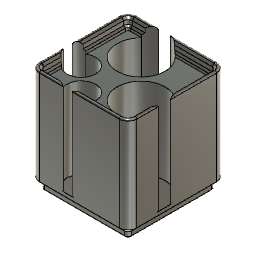
Gridfinity CR2032 + LR44 Holder (Autodesk Fusion 360 design; units mm, degrees)
Autodesk Fusion 360 part; units mm, degrees
sketch "Sketch1" plane through (0, 0, 0) normal (0, 0, 1) x (1, 0, 0) in component "Blank Storage"
  line L0 (0, 42) -> (42, 42)
  line L1 (42, 42) -> (42, 0)
  line L2 (42, 0) -> (0, 0)
  line L3 (0, 0) -> (0, 42)
  line L4 (0, 42) -> (42, 0) construction
  line L5 (42, 21) -> (0, 21) construction
  line L6 (42, 14.5) -> (0, 14.5)
  line L7 (42, 27.5) -> (0, 27.5)
  line L8 (27.5, 42) -> (27.5, 0)
  line L9 (14.5, 42) -> (14.5, 0)
  line L10 (14.5, 14.5) -> (0, 0) construction
  circle A0 centre (8, 8) radius 1.5
  circle A1 centre (34, 8) radius 1.5
  circle A2 centre (34, 34) radius 1.5
  circle A3 centre (8, 34) radius 1.5
  circle A4 centre (8, 8) radius 3.25
  circle A5 centre (34, 8) radius 3.25
  circle A6 centre (34, 34) radius 3.25
  circle A7 centre (8, 34) radius 3.25
  point P0 (21, 21)
  dimension "d1" = 42
  dimension "d2" = 42
  dimension "d65" = 13
  dimension "d67" = 90
  dimension "d69" = 3
  dimension "d71" = 360
  dimension "d80" = 6.5
  dimension "d85" = 8
  constraint horizontal L0
  constraint perpendicular L0 L1
  constraint parallel L0 L2
  constraint parallel L1 L3
  constraint coincident L2.end L3.start
  constraint midpoint L1 L5.start
  constraint midpoint L3 L5.end
  constraint coincident L1 L6.start
  constraint coincident L3 L6.end
  constraint perpendicular L3 L6
  constraint symmetric L5 L6.start L7.start
  constraint symmetric L5 L6.end L7.end
  constraint midpoint L4 P0
  constraint coincident L9 L10.start
  constraint coincident L6 L10.start
  constraint concentric A0 A4
  constraint coincident L10 A0.centre
  measures "d1" distance of L1.end L2.end
  measures "d2" distance of L0.end L1.end
  measures "d65" distance of L6 L7
  measures "d69" diameter of A0
  measures "d80" diameter of A4
  measures "d85" distance of L2 A0.centre
extrude "Extrude1" add sketch "Sketch1" along normal blind 5 contours L0 L3 L7 L9 | L0 L7 L8 L9 | L3 L6 L7 L9 | L0 L1 L7 L8 | L6 L7 L8 L9 | L2 L3 L6 L9 | L1 L6 L7 L8 | L2 L6 L8 L9 | L1 L2 L6 L8 | A0 | A1 | A2 | A3 | A4 | A5 | A6 | A7 makes body 1 in component "Blank Storage"
ref_plane "WorkPlane1" through (21, 21, 2.5) normal (0, -1, 0) x (1, 0, 0) in component "Blank Storage"
sketch "Sketch2" plane through (0, 21, 0) normal (0, -1, 0) x (1, 0, 0) in component "Blank Storage"
  line L0 (42, 0) -> (0, 0)
  line L1 (0, 0) -> (0, 5)
  line L2 (3.2, 0) -> (2.4, 0.8)
  line L3 (3.2, 0) -> (0, 0) construction
  line L4 (2.4, 0.8) -> (2.4, 2.6)
  line L5 (2.4, 2.6) -> (0, 5)
  line L6 (0, 5) -> (-5.1222, 5)
  line L7 (-5.1222, 5) -> (-5.1222, -0.0937)
  line L8 (-5.1222, -0.0937) -> (0, 0)
  dimension "d39" = 45
  dimension "d40" = 45
  dimension "d41" = 0.8
  dimension "d43" = 5
  dimension "d112" = 2.4
  constraint horizontal L3
  constraint coincident L0 L2.start
  constraint perpendicular L0 L4
  constraint coincident L1 L5.end
  constraint coincident L0.end L1.start
  constraint coincident L1.end L5.end
  constraint perpendicular L1 L6
  constraint perpendicular L6 L7
  measures "d39" angle of L2 L3
  measures "d40" angle of L4 L5
  measures "d41" distance of L2.end L3
  measures "d43" distance of L3 L1.end
  measures "d112" horizontal distance of L0.end L2.end
sketch "Sketch3" plane through (0, 0, 0) normal (0, 0, -1) x (1, 0, 0)
  line L0 (42, 0) -> (0, 0)
  line L1 (0, 0) -> (0, -42)
  line L2 (0, -42) -> (42, -42)
  line L3 (42, -42) -> (42, 0)
  arc A0 (4, 0) -> (0, -4) centre (4, -4) ccw
  line L4 (0, -42) -> (42, 0) construction
  arc A1 (0, -38) -> (4, -42) centre (4, -38) ccw
  arc A2 (38, -42) -> (42, -38) centre (38, -38) ccw
  arc A3 (42, -4) -> (38, 0) centre (38, -4) ccw
  line L5 (0, -4) -> (0, -38)
  line L6 (4, -42) -> (38, -42)
  line L7 (42, -38) -> (42, -4)
  line L8 (38, 0) -> (4, 0)
  point P0 (21, -21)
  dimension "d37" = 360
  constraint coincident L1.end L2.start
  constraint coincident L0.start L3.end
  constraint midpoint L4 P0
sweep "Sweep1" cut profiles "Sketch2" path "Sketch3" along L8 A0 L5 A1 L6 A2 L7 A3 section 1 bodies 1 in component "Blank Storage"
extrude "Extrude1'" add sketch "Sketch3" against normal up to surface (5 mm away) separate body makes body 2 in component "Blank Frame"
combine "Combine1" operation cut target body 2 tool bodies 1 keep tools in component "Blank Frame"
move_face "OffsetFaces1" offset -0.25 24 faces at (40.4, 26.6667, 3.4) (40.6565, 38.2324, 3.6667) (39.1041, 39.158, 2) (15.3333, 39.0667, 0.2667) (39.2397, 38.1085, 0.4444) (26.6667, 39.6, 1.4) (26.6667, 40.4, 3.4) (39.6, 15.3333, 1.4) (39.0667, 15.3333, 0.2667) (38.2324, 1.3435, 3.6667) (3.7676, 40.6565, 3.6667) (3.9239, 39.5982, 1.4) (3.8915, 39.2397, 0.4444) (2.4, 26.6667, 1.4) (2.9333, 15.3333, 0.2667) (1.6, 26.6667, 3.4) (1.3435, 3.7676, 3.6667) (2.4018, 3.9239, 1.4) (2.7603, 3.8915, 0.4444) (15.3333, 2.4, 1.4) (15.3333, 2.9333, 0.2667) (15.3333, 0.8, 4.2) (39.2397, 3.8915, 0.4444) (39.158, 2.8959, 1.4) on bodies 2 in component "Blank Frame"
extrude "Extrude3" [suppressed] in component "Blank Storage"
draft "Draft1" [suppressed] in component "Blank Storage"
extrude "Extrude4" cut sketch "Sketch1" along normal up to surface (5 mm away) contours A0 | A1 | A2 | A3 bodies 1 in component "Blank Storage"
extrude "Extrude5" cut sketch "Sketch1" along normal blind 2.4 contours A4 | A5 | A6 | A7 bodies 1 in component "Blank Storage"
pattern_linear "R-Pattern1" count 1 spacing 42 along (1, 0, 0) of bodies 1 merged in component "Blank Storage"
sketch "Sketch4" plane through (0, 0, 5) normal (0, 0, 1) x (-1, 0, 0) in component "Blank Storage"
  line L0 (-4, 0) -> (-38, 0)
  line L1 (-42, -4) -> (-42, -38)
  line L2 (-38, -42) -> (-4, -42)
  line L3 (0, -38) -> (0, -4)
  arc A0 (0, -4) -> (-4, 0) centre (-4, -4) ccw
  arc A1 (-38, 0) -> (-42, -4) centre (-38, -4) ccw
  arc A2 (-42, -38) -> (-38, -42) centre (-38, -38) ccw
  arc A3 (-4, -42) -> (0, -38) centre (-4, -38) ccw
  line L4 (-38, -41.75) -> (-4, -41.75)
  arc A4 (-4, -41.75) -> (-0.25, -38) centre (-4, -38) ccw
  line L5 (-0.25, -38) -> (-0.25, -4)
  arc A5 (-0.25, -4) -> (-4, -0.25) centre (-4, -4) ccw
  line L6 (-4, -0.25) -> (-38, -0.25)
  arc A6 (-38, -0.25) -> (-41.75, -4) centre (-38, -4) ccw
  line L7 (-41.75, -4) -> (-41.75, -38)
  arc A7 (-41.75, -38) -> (-38, -41.75) centre (-38, -38) ccw
  point P0 (-42, 0)
  point P1 (0, -42)
  dimension "d44" = 42
  dimension "d45" = 42
  dimension "d48" = 4
  dimension "d49" = 4
  dimension "d50" = 4
  dimension "d51" = 4
  dimension "d118" = -0.25
  constraint horizontal L0
  constraint vertical L1
  constraint horizontal L2
  constraint vertical L3
  constraint coincident origin L0
  constraint coincident origin L3
  constraint tangent L0 A0
  constraint tangent L3 A0
  constraint coincident P0 L0
  constraint coincident P0 L1
  constraint tangent L0 A1
  constraint tangent L1 A1
  constraint tangent L1 A2
  constraint tangent L2 A2
  constraint coincident P1 L2
  constraint coincident P1 L3
  constraint tangent L2 A3
  constraint tangent L3 A3
  measures "d44" distance of origin P0
  measures "d45" distance of origin P1
  measures "d48" radius of A0
  measures "d49" radius of A1
  measures "d50" radius of A2
  measures "d51" radius of A3
extrude "Extrude2" add sketch "Sketch4" along normal blind 37 contours L0 L1 L2 L3 A0 A1 A2 A3 | L4 A4 L5 A5 L6 A6 L7 A7 bodies 1 in component "Blank Storage"
sketch "Sketch5" plane through (21, 21, 2.5) normal (0, -1, 0) x (1, 0, 0) in component "Blank Storage"
  line L0 (-18.6, 0.1) -> (-21, 2.5)
  line L1 (17, 2.5) -> (-17, 2.5)
  line L2 (-18.6, -1.7) -> (-18.6, 0.1)
  line L3 (-17.8, -2.5) -> (-18.6, -1.7)
  line L4 (-17, 39.5) -> (-21, 39.5)
  line L5 (-17, 39.5) -> (-21, 39.5)
  line L6 (-17, 39.5) -> (17, 39.5)
  line L7 (21, 39.5) -> (17, 39.5)
  line L8 (21, 39.5) -> (17, 39.5)
  line L9 (17, 39.5) -> (-17, 39.5)
  line L10 (-18.6, 42.1) -> (-21, 44.5)
  line L11 (-18.6, 40.3) -> (-18.6, 42.1)
  line L12 (-17.8, 39.5) -> (-18.6, 40.3)
  line L13 (-21, 2.5) -> (-21, 39.5)
  line L14 (-21, 39.5) -> (-21, 2.5)
  line L15 (-17.8, 39.5) -> (-21, 39.5)
  line L16 (-21, 44.5) -> (-21, 39.5)
  line L17 (-17.9768, 39.3232) -> (-18.85, 40.1964)
  line L18 (-18.85, 40.1964) -> (-18.85, 41.9964)
  line L19 (-18.85, 41.9964) -> (-21.1768, 44.3232)
  dimension "d54" = 0
  dimension "d55" = 42
  dimension "d131" = 4.8232
  constraint coincident L14 L4.end
  constraint perpendicular L14 L15
  measures "d131" vertical distance of L4.end L19.end
sweep "Sweep2" add profiles "Sketch5" along 8 edges at (21, 0, 42) (40.8284, 1.1716, 42) (42, 21, 42) (40.8284, 40.8284, 42) (21, 42, 42) (1.1716, 40.8284, 42) (0, 21, 42) (1.1716, 1.1716, 42) section 1 contours L4 L5 L15 L16 L17 L18 L19 on bodies 1 bodies 1 in component "Blank Storage"
extrude "Extrude2'" cut sketch "Sketch4" along normal through all and the other way through all bodies 1 in component "Blank Storage"
fillet "Fillet2" radius 0.6 8 edges at (21, 0.25, 46.3964) (40.6517, 1.3483, 46.3964) (41.75, 21, 46.3964) (40.6517, 40.6517, 46.3964) (21, 41.75, 46.3964) (1.3483, 40.6517, 46.3964) (0.25, 21, 46.3964) (1.3483, 1.3483, 46.3964) on bodies 1 in component "Blank Storage"
extrude "Extrude1''" cut 1 faces at (27.0512, 15.3333, 42) along direction (0, 0, -1) up to surface (35.8 mm away) on bodies 1 bodies 1 in component "Blank Storage"
extrude "Extrude3'" add 1 faces at (27.0512, 15.3333, 6.2) along direction (0, 0, 1) blind 34.65 separate body on bodies 1 makes body 3 in component "Blank Storage"
sketch "Sketch7" plane through (0, 0, 6.2) normal (0, 0, 1) x (-1, 0, 0)
  line L0 (-2.8464, -38) -> (-2.8464, -4)
  arc A0 (-2.8464, -4) -> (-4, -2.8464) centre (-4, -4) ccw
  line L1 (-4, -2.8464) -> (-38, -2.8464)
  arc A1 (-38, -2.8464) -> (-39.1536, -4) centre (-38, -4) ccw
  line L2 (-39.1536, -4) -> (-39.1536, -38)
  arc A2 (-39.1536, -38) -> (-38, -39.1536) centre (-38, -38) ccw
  line L3 (-38, -39.1536) -> (-4, -39.1536)
  arc A3 (-4, -39.1536) -> (-2.8464, -38) centre (-4, -38) ccw
  circle A4 centre (-15.7995, -31.8) radius 10.25
  line L4 (0, 0) -> (-41.7996, -41.7996) construction
  circle A5 centre (-31.8, -15.7995) radius 10.25
  circle A6 centre (-6.075, -16) radius 6.125
  circle A7 centre (-16, -6.075) radius 6.125
  line L5 (-0.25, -4) -> (-0.25, -38)
  line L6 (-4, -41.75) -> (-38, -41.75)
  dimension "d122" = 20.5
  dimension "d124" = 12.25
  dimension "d129" = 5.825
  dimension "d130" = 9.95
  constraint coincident L4.start origin
  constraint symmetric A4 L4 A5
  constraint symmetric L4 A6 A7
  measures "d122" diameter of A4
  measures "d124" diameter of A6
  measures "d129" distance of A6.centre L5
  measures "d130" distance of A4.centre L6
extrude "Extrude4'" cut sketch "Sketch7" along normal blind 40 contours L0 A6 | L0 A6 L5 | A6 L5 | L3 A4 L6 | L3 A4 | A4 L6 | L1 A7 | L1 A7 | L2 A5 | L2 A5 bodies 1 3 in component "Blank Storage"
sketch "Skizze8" plane through (0, 0, 40.85) normal (0, 0, 1) x (-1, 0, 0)
  arc A0 (-2.8464, -10.795) -> (-2.8464, -21.205) centre (-6.075, -16) ccw
  line L0 (-2.8464, -10.795) -> (-2.8464, -4)
  arc A1 (-2.8464, -4) -> (-4, -2.8464) centre (-4, -4) ccw
  line L1 (-4, -2.8464) -> (-10.795, -2.8464)
  arc A2 (-21.205, -2.8464) -> (-10.795, -2.8464) centre (-16, -6.075) ccw
  line L2 (-21.205, -2.8464) -> (-38, -2.8464)
  arc A3 (-38, -2.8464) -> (-39.1536, -4) centre (-38, -4) ccw
  line L3 (-39.1536, -4) -> (-39.1536, -8.659)
  arc A4 (-39.1536, -22.9401) -> (-39.1536, -8.659) centre (-31.8, -15.7995) ccw
  line L4 (-39.1536, -22.9401) -> (-39.1536, -38)
  arc A5 (-39.1536, -38) -> (-38, -39.1536) centre (-38, -38) ccw
  line L5 (-38, -39.1536) -> (-22.9401, -39.1536)
  arc A6 (-8.659, -39.1536) -> (-22.9401, -39.1536) centre (-15.7995, -31.8) ccw
  line L6 (-8.659, -39.1536) -> (-4, -39.1536)
  arc A7 (-4, -39.1536) -> (-2.8464, -38) centre (-4, -38) ccw
  line L7 (-2.8464, -38) -> (-2.8464, -21.205)
component "Blank Storage" placed x (1, 0, 0) y (0, 1, 0) z (0, 0, 1) at (0, 0, 0)
component "Blank Frame" placed x (1, 0, 0) y (0, 1, 0) z (0, 0, 1) at (0, 0, 0)
equation "d1 = slotDimension"
equation "d2 = slotDimension"
equation "d3 = nestingDepth"
equation "slotsWide = 1"
equation "slotsHigh = 1"
equation "slotsDeep = 1"
equation "slotDimension = 42 mm"
equation "nestingDepth = 5 mm"
equation "nestingRimWidth = 2.4 mm"
equation "nestingClearance = 0.25 mm"
equation "cornerFillet = 4 mm"
equation "d31 = slotsWide"
equation "d32 = slotsDeep"
equation "d33 = slotDimension"
equation "d34 = slotDimension"
equation "d38 = -slotDimension / 2"
equation "d43 = nestingDepth"
equation "d44 = slotDimension * slotsWide"
equation "d45 = slotDimension * slotsDeep"
equation "d46 = slotDimension * slotsHigh - nestingDepth"
equation "d48 = cornerFillet"
equation "d49 = cornerFillet"
equation "d50 = cornerFillet"
equation "d51 = cornerFillet"
equation "d55 = slotDimension * slotsHigh"
equation "d56 = -nestingClearance"
equation "ledStripWidth = 13 mm"
equation "ledSlotHeight = 4 mm"
equation "d65 = ledStripWidth"
equation "screwTightDiameter = 3 mm"
equation "d69 = screwTightDiameter"
equation "d72 = ledSlotHeight"
equation "magnetDiameter = 6.5 mm"
equation "magnetThiccness = 2.4 mm"
equation "d80 = magnetDiameter"
equation "d81 = magnetThiccness"
equation "d90 = -nestingClearance"
equation "d98 = -wallThiccness"
equation "wallThiccness = 1.2 mm"
equation "d112 = nestingRimWidth"
equation "d122 = 20 mm + BatteryClearance"
equation "d124 = 11.75 mm + BatteryClearance"
equation "d125 = slotDimension * slotsHigh * 0.95 - nestingDepth - nestingClearance"
equation "d129 = d124 / 2 - BatteryBoxOverhang"
equation "d130 = d122 / 2 - BatteryBoxOverhang"
equation "BatteryClearance = 0.5 mm"
equation "BatteryBoxOverhang = 0.3 mm"
